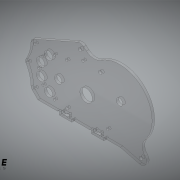
# Autodesk Inventor part: アームフレーム改
Saved by Autodesk Inventor 2020 (Build 240168000, 168)
## iProperties
Created: 2019-12-31
Part Number: アームフレーム改
Material: ポリカーボネート、クリア
Document SubType Name: Modeling
Designer: tanjihayato
Density: 1.2 g/cm^3
Appearance: ポリカーボネート - クリア
Author: tanjihayato
Autodesk Inventor part; units mm, degrees
ref_plane "YZ Plane" through (0, 0, 0) normal (1, 0, 0) x (0, 1, 0)
ref_plane "XZ Plane" through (0, 0, 0) normal (0, 1, 0) x (-1, 0, 0)
ref_plane "XY Plane" through (0, 0, 0) normal (0, 0, 1) x (1, 0, 0)
sketch "スケッチ2" plane through (0, 0, 0) normal (0, 0, 1) x (1, 0, 0)
  circle A0 centre (54.047, 13.5882) radius 4.025
  circle A1 centre (80.4159, -30.3183) radius 2
  circle A2 centre (30.7326, 32.4678) radius 2
  circle A3 centre (3.7003, 45.5208) radius 2
  circle A4 centre (8.8763, 3.8907) radius 7.5
  circle A5 centre (-39.4931, -19.1593) radius 5
  circle A6 centre (-49.0547, -7.5196) radius 5
  circle A7 centre (-49.0547, 7.5438) radius 5
  circle A8 centre (-39.4931, 19.1835) radius 5
  circle A9 centre (-28.0204, 0.0121) radius 4.5
  circle A10 centre (-5.4761, 38.5895) radius 1.5
  circle A11 centre (69.7531, -26.0108) radius 1.5
  circle A12 centre (12.7384, 41.2415) radius 1.5
  circle A13 centre (-56.0504, -23.0135) radius 1.5
  circle A14 centre (-16.1798, -24.0771) radius 1.5
  circle A15 centre (-64.2952, 0.0121) radius 1.5
  circle A16 centre (-56.0504, 23.0377) radius 1.5
  circle A17 centre (-21.4477, 26.0369) radius 1.5
  circle A18 centre (34.0114, -24.0061) radius 1.5
  circle A19 centre (-32.6283, -23.2673) radius 1.3
  circle A20 centre (-46.3578, -15.0513) radius 1.3
  circle A21 centre (-51.7515, 0.0121) radius 1.3
  circle A22 centre (-46.3578, 15.0755) radius 1.3
  circle A23 centre (-32.6283, 23.2915) radius 1.3
  line L0 (-24.5547, -30.1593) -> (-24.5547, -33.1593)
  arc A24 (-26.6547, -33.1593) -> (-24.5547, -33.1593) centre (-25.6047, -33.1593) ccw
  line L1 (-26.6547, -33.1593) -> (-31.4547, -33.1593)
  arc A25 (-33.5547, -33.1593) -> (-31.4547, -33.1593) centre (-32.5047, -33.1593) ccw
  line L2 (-33.5547, -33.1593) -> (-33.5547, -30.1593)
  arc A26 (-31.4547, -30.1593) -> (-33.5547, -30.1593) centre (-32.5047, -30.1593) ccw
  line L3 (-31.4547, -30.1593) -> (-26.6547, -30.1593)
  arc A27 (-24.5547, -30.1593) -> (-26.6547, -30.1593) centre (-25.6047, -30.1593) ccw
  line L4 (13.9305, -30.1593) -> (13.9305, -33.1593)
  arc A28 (11.8305, -33.1593) -> (13.9305, -33.1593) centre (12.8805, -33.1593) ccw
  line L5 (11.8305, -33.1593) -> (7.0305, -33.1593)
  arc A29 (4.9305, -33.1593) -> (7.0305, -33.1593) centre (5.9805, -33.1593) ccw
  line L6 (4.9305, -33.1593) -> (4.9305, -30.1593)
  arc A30 (7.0305, -30.1593) -> (4.9305, -30.1593) centre (5.9805, -30.1593) ccw
  line L7 (7.0305, -30.1593) -> (11.8305, -30.1593)
  arc A31 (13.9305, -30.1593) -> (11.8305, -30.1593) centre (12.8805, -30.1593) ccw
  arc A32 (19.0305, -33.1593) -> (16.9305, -33.1593) centre (17.9805, -33.1593) ccw
  line L8 (19.0305, -33.1593) -> (56.2168, -33.1593)
  line L9 (56.2168, -33.1593) -> (79.2003, -37.212)
  arc A33 (79.2003, -37.212) -> (87.3507, -31.2711) centre (80.4159, -30.3183) ccw
  line L10 (87.3507, -31.2711) -> (92.7831, 8.2659)
  arc A34 (92.7831, 8.2659) -> (29.742, 44.2162) centre (54.047, 13.5882) ccw
  arc A35 (15.9809, 44.3871) -> (29.742, 44.2162) centre (22.9664, 52.7545) ccw
  line L11 (15.9809, 44.3871) -> (8.1864, 50.8943)
  arc A36 (8.1864, 50.8943) -> (0.9804, 51.9708) centre (3.7003, 45.5208) ccw
  line L12 (0.9804, 51.9708) -> (-67.2952, 23.1796)
  line L13 (-67.2952, 23.1796) -> (-67.2952, -18.1327)
  line L14 (-67.2952, -18.1327) -> (-52.2685, -33.1593)
  line L15 (-52.2685, -33.1593) -> (-38.6547, -33.1593)
  arc A37 (-36.5547, -33.1593) -> (-38.6547, -33.1593) centre (-37.6047, -33.1593) ccw
  line L16 (-36.5547, -33.1593) -> (-36.5547, -36.1593)
  line L17 (-36.5547, -36.1593) -> (-21.5547, -36.1593)
  line L18 (-21.5547, -36.1593) -> (-21.5547, -33.1593)
  arc A38 (-19.4547, -33.1593) -> (-21.5547, -33.1593) centre (-20.5047, -33.1593) ccw
  line L19 (-19.4547, -33.1593) -> (-0.1695, -33.1593)
  arc A39 (1.9305, -33.1593) -> (-0.1695, -33.1593) centre (0.8805, -33.1593) ccw
  line L20 (1.9305, -33.1593) -> (1.9305, -36.1593)
  line L21 (1.9305, -36.1593) -> (16.9305, -36.1593)
  line L22 (16.9305, -36.1593) -> (16.9305, -33.1593)
  point P0 (0, 0)
  point P1 (0, 0)
  constraints: 46 end point, 40 centre point, 32 point on circle
sketch "スケッチ1" plane through (0, 0, 0) normal (0, 0, 1) x (1, 0, 0)
  line L0 (-170.6512, -31.4118) -> (202.8656, -31.4118) construction
  circle A0 centre (-14, -17.4118) radius 14 construction
  circle A1 centre (14, -17.4118) radius 14 construction
  circle A2 centre (-28.0204, 0.0121) radius 20.05 construction
  circle A3 centre (-28.0204, 0.0121) radius 5.05 construction
  circle A4 centre (5.5774, 0.3907) radius 28.55 construction
  circle A5 centre (5.5774, 0.3907) radius 10.1 construction
  circle A6 centre (45.6606, 13.5882) radius 32.1 construction
  line L1 (-170.915, -81.4118) -> (490.0044, -81.4118)
  circle A7 centre (-28.0204, 0.0121) radius 22.342 construction
  circle A8 centre (-39.4931, 19.1835) radius 14 construction
  circle A9 centre (-49.0547, 7.5438) radius 14 construction
  circle A10 centre (-49.0547, -7.5196) radius 14 construction
  circle A11 centre (-39.4931, -19.1593) radius 14 construction
  circle A12 centre (5.5774, 0.3907) radius 29.55 construction
  circle A13 centre (45.6606, 13.5882) radius 34.1 construction
  line L2 (-67.2952, 44.8622) -> (-67.2952, -57.3934) construction
  line L3 (-149.4523, -1.6098) -> (-132.6633, -31.6026)
  line L4 (-132.7701, -31.4118) -> (-132.7701, 74.0456)
  circle A14 centre (-11.4931, -19.1593) radius 14 construction
  line L5 (-197.2268, -33.1593) -> (179.6604, -33.1593) construction
  circle A15 centre (45.6606, 13.5882) radius 4.025
  circle A16 centre (45.6606, 13.5882) radius 6
  circle A17 centre (-39.4931, 19.1835) radius 5
  circle A18 centre (-49.0547, 7.5438) radius 5
  circle A19 centre (-49.0547, -7.5196) radius 5
  circle A20 centre (-39.4931, -19.1593) radius 5
  circle A21 centre (-39.4931, 19.1835) radius 8 construction
  circle A22 centre (-49.0547, 7.5438) radius 8 construction
  circle A23 centre (-49.0547, -7.5196) radius 8 construction
  circle A24 centre (-39.4931, -19.1593) radius 8 construction
  circle A25 centre (-28.0204, 0.0121) radius 4.5
  circle A26 centre (5.5774, 0.3907) radius 7.5
  line L6 (-17.5497, 32.3149) -> (-46.3578, 15.0755) construction
  line L7 (-46.3578, 15.0755) -> (-51.7515, 0.0121) construction
  line L8 (-51.7515, 0.0121) -> (-46.3578, -15.0513) construction
  line L9 (-46.3578, -15.0513) -> (-37.9391, -20.0892) construction
  circle A27 centre (-32.6283, 23.2915) radius 1.3
  circle A28 centre (-46.3578, 15.0755) radius 1.3
  circle A29 centre (-51.7515, 0.0121) radius 1.3
  circle A30 centre (-46.3578, -15.0513) radius 1.3
  circle A31 centre (-32.6283, -23.2673) radius 1.3
  line L10 (-67.2952, 23.0074) -> (-67.2952, -18.1327)
  arc A32 (69.4805, -38.9096) -> (76.2418, -27.2762) centre (71.1898, -32.1215) ccw
  arc A33 (2.6419, 49.4236) -> (-4.7411, 50.524) centre (-1.9226, 44.1165) ccw
  line L11 (-52.2685, -33.1593) -> (46.6439, -33.1593)
  line L12 (46.6439, -33.1593) -> (69.4805, -38.9096)
  arc A34 (75.6915, -11.451) -> (23.3358, 45.6882) centre (45.6606, 13.5882) ccw
  line L13 (-4.7411, 50.524) -> (-67.2952, 23.0074)
  circle A35 centre (31.0922, -22.157) radius 4.5 construction
  circle A36 centre (31.0922, -22.157) radius 1.5
  circle A37 centre (-18.0319, 24.9264) radius 4.5 construction
  circle A38 centre (-18.0319, 24.9264) radius 1.5
  circle A39 centre (-56.0504, 23.0377) radius 1.5
  circle A40 centre (-56.0504, 23.0377) radius 3 construction
  circle A41 centre (-56.0504, 23.0377) radius 4.5 construction
  circle A42 centre (-64.2952, 0.0121) radius 1.5
  circle A43 centre (-64.2952, 0.0121) radius 3 construction
  circle A44 centre (-64.2952, 0.0121) radius 4.3311 construction
  line L14 (45.6606, 13.5882) -> (91.8641, 32.6996) construction
  line L15 (91.8641, 32.6996) -> (51.4166, 12.9764) construction
  line L16 (51.4166, 12.9764) -> (22.3463, 32.4678) construction
  line L17 (22.3463, 32.4678) -> (45.6606, 13.5882) construction
  line L18 (91.8641, 32.6996) -> (455.8912, 210.2081)
  line L19 (-183.2789, 162.2213) -> (-183.2789, -125.2315)
  line L20 (516.7211, 155.5913) -> (516.7211, -155.5644)
  circle A45 centre (91.8641, 32.6996) radius 7.25
  line L21 (127.8174, 50.2313) -> (416.2031, 132.8973) construction
  line L22 (224.3644, 77.9066) -> (174.0148, 126.537) construction
  circle A46 centre (-1.9226, 44.1165) radius 4
  circle A47 centre (114.3349, 43.6569) radius 2
  circle A48 centre (127.8174, 50.2313) radius 2
  arc A49 (130.5797, 46.0636) -> (126.2347, 54.9742) centre (127.8174, 50.2313) ccw
  line L23 (130.5797, 46.0636) -> (97.5269, 24.1559)
  line L24 (126.2347, 54.9742) -> (88.6196, 42.4225)
  circle A50 centre (22.3463, 32.4678) radius 2
  circle A51 centre (-17.4731, -24.6708) radius 4.5 construction
  circle A52 centre (-17.4731, -24.6708) radius 1.5
  line L25 (-67.2952, -18.1327) -> (-52.2685, -33.1593)
  circle A53 centre (-56.0504, -23.0135) radius 1.5
  circle A54 centre (-56.0504, -23.0135) radius 3 construction
  circle A55 centre (22.3463, 32.4678) radius 4 construction
  arc A56 (45.9958, 17.0721) -> (45.5027, 10.0918) centre (45.6606, 13.5882) ccw construction
  line L26 (88.9298, 31.4858) -> (92.2801, 35.8476) construction
  line L27 (92.2801, 35.8476) -> (94.3823, 30.7652) construction
  line L28 (94.3823, 30.7652) -> (88.9298, 31.4858) construction
  circle A57 centre (94.3823, 30.7652) radius 1.5
  circle A58 centre (92.2801, 35.8476) radius 1.5
  circle A59 centre (88.9298, 31.4858) radius 1.5
  circle A60 centre (91.8641, 32.6996) radius 6
  arc A61 (96.9465, 25.8864) -> (84.4967, 36.9388) centre (91.8641, 32.6996) ccw
  arc A62 (45.9958, 17.0721) -> (84.4967, 36.9388) centre (49.8265, 56.8883) ccw construction
  arc A63 (45.5027, 10.0918) -> (96.9465, 25.8864) centre (49.1121, 90.0103) ccw construction
  circle A64 centre (45.6606, 13.5882) radius 8.5 construction
  line L29 (88.6151, 40.5541) -> (42.4117, 21.4428) construction
  line L30 (48.9096, 5.7336) -> (95.113, 24.845) construction
  circle A65 centre (71.1898, -32.1215) radius 4
  circle A66 centre (-56.0504, -23.0135) radius 4.5 construction
  line L31 (2.6419, 49.4236) -> (5.9468, 46.5813)
  circle A67 centre (1.6221, 34.2101) radius 1.5
  circle A68 centre (1.6221, 34.2101) radius 4.5 construction
  circle A69 centre (45.6606, 13.5882) radius 50 construction
  circle A70 centre (-1.9226, 44.1165) radius 2
  circle A71 centre (71.1898, -32.1215) radius 2
  circle A72 centre (45.6606, 13.5882) radius 1.5 construction
  circle A73 centre (51.4166, 12.9764) radius 1.5 construction
  circle A74 centre (51.4166, 12.9764) radius 3 construction
  circle A75 centre (51.4166, 12.9764) radius 5 construction
  line L32 (95.251, 23.0253) -> (53.0688, 8.2573) construction
  line L33 (48.7158, 17.1842) -> (86.3274, 41.3256) construction
  arc A76 (88.6196, 42.4225) -> (86.3274, 41.3256) centre (91.8641, 32.6996) ccw
  arc A77 (95.251, 23.0253) -> (97.5269, 24.1559) centre (91.8641, 32.6996) ccw
  circle A78 centre (22.3463, 32.4678) radius 5.025 construction
  circle A79 centre (22.3463, 32.4678) radius 8.025 construction
  circle A80 centre (51.4166, 12.9764) radius 4.025 construction
  circle A81 centre (51.4166, 12.9764) radius 7.025 construction
  line L34 (18.0694, 25.6774) -> (47.6727, 7.0322) construction
  line L35 (46.0495, 17.5091) -> (29.1233, 28.1698) construction
  line L36 (58.3798, 13.9061) -> (60.365, -0.9619) construction
  line L37 (60.365, -0.9619) -> (47.6727, 7.0322) construction
  arc A82 (5.9468, 46.5813) -> (23.3358, 45.6882) centre (15.2178, 57.3607) ccw
  circle A83 centre (5.5774, 0.3907) radius 12.1 construction
  circle A84 centre (-28.0204, 0.0121) radius 20.55 construction
  line L38 (-10.1028, -29.1593) -> (39.2109, -29.1593) construction
  arc A85 (75.6915, -11.451) -> (76.2418, -27.2762) centre (84.8125, -19.056) ccw
  line L39 (-36.5547, -36.1593) -> (-21.5547, -36.1593) projected
  line L40 (1.9305, -36.1593) -> (16.9305, -36.1593) projected
  line L41 (-26.5547, -36.1593) -> (-11.5547, -36.1593)
  line L42 (11.9305, -36.1593) -> (26.9305, -36.1593)
  line L43 (-26.5547, -36.1593) -> (-26.5547, -33.1593)
  line L44 (11.9305, -36.1593) -> (11.9305, -33.1593)
  line L45 (26.9305, -36.1593) -> (26.9305, -33.1593)
  line L46 (-11.5547, -36.1593) -> (-11.5547, -33.1593)
  point P0 (0, 0)
  point P1 (0, 0)
  point P2 (-49.0547, 7.5438)
  point P3 (-49.0547, -7.5196)
  dimension "d0" = 40.1
  dimension "d1" = 10.1
  dimension "d2" = 20.2
  dimension "d3" = 95
  dimension "d4" = 44.684
  dimension "d5" = 28
  dimension "d6" = 28
  dimension "d7" = 28
  dimension "d8" = 28
  dimension "d9" = 1
  dimension "d10" = 2
  dimension "d11" = 8.05
  dimension "d12" = 12
  dimension "d13" = 10
  dimension "d14" = 10
  dimension "d15" = 10
  dimension "d16" = 10
  dimension "d17" = 3
  dimension "d18" = 3
  dimension "d19" = 3
  dimension "d20" = 3
  dimension "d21" = 9
  dimension "d22" = 15
  dimension "d23" = 2.6
  dimension "d24" = 2.6
  dimension "d25" = 2.6
  dimension "d26" = 2.6
  dimension "d27" = 2.6
  dimension "d28" = 5
  dimension "d29" = 9
  dimension "d30" = 3
  dimension "d31" = 9
  dimension "d32" = 3
  dimension "d33" = 3
  dimension "d34" = 6
  dimension "d35" = 9
  dimension "d36" = 3
  dimension "d37" = 6
  dimension "d38" = 50
  dimension "d39" = 45
  dimension "d40" = 35
  dimension "d41" = 30
  dimension "d42" = 39
  dimension "d43" = 700
  dimension "d44" = 14.5
  dimension "d45" = 300
  dimension "d46" = 10
  dimension "d47" = 70
  dimension "d48" = 120
  dimension "d49" = 140
  dimension "d50" = 8
  dimension "d51" = 4
  dimension "d52" = 4
  dimension "d53" = 15
  dimension "d54" = 25
  dimension "d55" = 10
  dimension "d56" = 4
  dimension "d57" = 9
  dimension "d58" = 3
  dimension "d59" = 3
  dimension "d60" = 6
  dimension "d61" = 45
  dimension "d62" = 8
  dimension "d63" = 7
  constraints: 90 end point, 83 centre point, 53 tangent, 44 coincident, 41 point on circle, 17 point on line, 7 vertical, 4 horizontal, 4 midpoint, 2 collinear, 1 parallel, 1 perpendicular, 1 vertical alignment, 18 other
  measures "d0" diameter of A2
  measures "d1" diameter of A3
  measures "d2" diameter of A5
  measures "d3" distance from line of L1 A6.centre
  measures "d4" diameter of A7
  measures "d5" diameter of A8
  measures "d6" diameter of A9
  measures "d7" diameter of A10
  measures "d8" diameter of A11
  measures "d9" radial gap between concentric circles of A4 A12
  measures "d10" radial gap between concentric circles of A6 A13
  measures "d11" diameter of A15
  measures "d12" diameter of A16
  measures "d13" diameter of A17
  measures "d14" diameter of A18
  measures "d15" diameter of A19
  measures "d16" diameter of A20
  measures "d17" radial gap between concentric circles of A17 A21
  measures "d21" diameter of A25
  measures "d22" diameter of A26
  measures "d23" diameter of A27
  measures "d24" diameter of A28
  measures "d25" diameter of A29
  measures "d26" diameter of A30
  measures "d27" diameter of A31
  measures "d28" radial gap between concentric circles of A13 A34
  measures "d29" diameter of A35
  measures "d30" diameter of A36
  measures "d31" diameter of A37
  measures "d32" diameter of A38
  measures "d33" diameter of A39
  measures "d34" diameter of A40
  measures "d35" diameter of A41
  measures "d36" diameter of A42
  measures "d37" diameter of A43
  measures "d38" distance of L14.start L14.end
  measures "d39" distance of L14.end L15.end
  measures "d40" distance of L15.end L16.end
  measures "d41" distance of L16.end L14.start
  measures "d42" angle of L0 L17
  measures "d43" distance between parallel lines of L20 L19
  measures "d44" diameter of A45
  measures "d45" distance of L21.start L21.end
  measures "d46" angle of L18 L21
  measures "d47" distance of L22.start L22.end
  measures "d48" angle of L21 L22
  measures "d49" distance of L14.end L22.start
  measures "d50" diameter of A46
  measures "d51" diameter of A47
  measures "d52" diameter of A48
  measures "d53" distance of L21.start A47.centre
  measures "d54" distance of A47.centre A45.centre
  measures "d55" diameter of A49
  measures "d56" diameter of A50
  measures "d57" diameter of A51
  measures "d58" diameter of A52
  measures "d59" diameter of A53
  measures "d60" diameter of A54
  measures "d61" angle of L5 L25
  measures "d62" diameter of A55
  measures "d63" diameter of A56
extrude "押し出し1" add sketch "スケッチ1" along normal blind 3 contours A16 | L13 A33 L31 A82 A34 A85 A32 L12 L11 L25 L10 | L11 L46 L41 L39 L43 | L11 L45 L42 L40 L44 | A46 | A65
sketch "スケッチ3" plane through (0, 0, 3) normal (0, 0, 1) x (1, 0, 0)
  line L0 (-52.2685, -33.1593) -> (-26.5547, -33.1593) projected
  line L1 (-26.5547, -33.1593) -> (-26.5547, -36.1593) projected
  line L2 (-26.5547, -36.1593) -> (-11.5547, -36.1593) projected
  line L3 (-11.5547, -36.1593) -> (-11.5547, -33.1593) projected
  line L4 (-11.5547, -33.1593) -> (11.9305, -33.1593) projected
  line L5 (11.9305, -33.1593) -> (11.9305, -36.1593) projected
  line L6 (11.9305, -36.1593) -> (26.9305, -36.1593) projected
  line L7 (26.9305, -36.1593) -> (26.9305, -33.1593) projected
  line L8 (26.9305, -33.1593) -> (46.6439, -33.1593) projected
  line L9 (46.6439, -33.1593) -> (69.4805, -38.9096) projected
  arc A0 (69.4805, -38.9096) -> (76.2418, -27.2762) centre (71.1898, -32.1215) ccw projected
  arc A1 (75.6915, -11.451) -> (76.2418, -27.2762) centre (84.8125, -19.056) ccw projected
  arc A2 (75.6915, -11.451) -> (23.3358, 45.6882) centre (45.6606, 13.5882) ccw projected
  arc A3 (5.9468, 46.5813) -> (23.3358, 45.6882) centre (15.2178, 57.3607) ccw projected
  line L10 (5.9468, 46.5813) -> (2.6419, 49.4236) projected
  arc A4 (2.6419, 49.4236) -> (-4.7411, 50.524) centre (-1.9226, 44.1165) ccw projected
  line L11 (-4.7411, 50.524) -> (-67.2952, 23.0074) projected
  line L12 (-67.2952, 23.0074) -> (-67.2952, -18.1327) projected
  line L13 (-67.2952, -18.1327) -> (-52.2685, -33.1593) projected
  circle A5 centre (-1.9226, 44.1165) radius 2 projected
  circle A6 centre (45.6606, 13.5882) radius 4.025 projected
  circle A7 centre (1.6221, 34.2101) radius 1.5 projected
  circle A8 centre (31.0922, -22.157) radius 1.5 projected
  circle A9 centre (-46.3578, -15.0513) radius 1.3 projected
  circle A10 centre (-46.3578, 15.0755) radius 1.3 projected
  circle A11 centre (5.5774, 0.3907) radius 7.5 projected
  circle A12 centre (-28.0204, 0.0121) radius 4.5 projected
  circle A13 centre (-39.4931, -19.1593) radius 5 projected
  circle A14 centre (-49.0547, -7.5196) radius 5 projected
  circle A15 centre (-49.0547, 7.5438) radius 5 projected
  circle A16 centre (-51.7515, 0.0121) radius 1.3 projected
  circle A17 centre (-32.6283, -23.2673) radius 1.3 projected
  circle A18 centre (-64.2952, 0.0121) radius 1.5 projected
  circle A19 centre (-17.4731, -24.6708) radius 1.5 projected
  circle A20 centre (22.3463, 32.4678) radius 2 projected
  circle A21 centre (-18.0319, 24.9264) radius 1.5 projected
  circle A22 centre (-56.0504, 23.0377) radius 1.5 projected
  circle A23 centre (-32.6283, 23.2915) radius 1.3 projected
  circle A24 centre (-56.0504, -23.0135) radius 1.5 projected
  circle A25 centre (-39.4931, 19.1835) radius 5 projected
  circle A26 centre (71.1898, -32.1215) radius 2 projected
  circle A27 centre (-56.0504, 23.0377) radius 4.5
  circle A28 centre (-64.2952, 0.0121) radius 3
  circle A29 centre (-56.0504, -23.0135) radius 4.5
  arc A30 (-66.8752, 1.5429) -> (-60.5479, 23.1875) centre (-105.8992, 24.6978) ccw
  arc A31 (-60.5479, -23.1633) -> (-66.8752, -1.5188) centre (-105.8992, -24.6736) ccw
  circle A32 centre (-49.0547, -7.5196) radius 14 construction
  circle A33 centre (-49.0547, 7.5438) radius 14 construction
  line L14 (-23.5547, -30.1593) -> (-14.5547, -30.1593)
  line L15 (-14.5547, -30.1593) -> (-14.5547, -33.1593)
  line L16 (-14.5547, -33.1593) -> (-23.5547, -33.1593)
  line L17 (-23.5547, -33.1593) -> (-23.5547, -30.1593)
  line L18 (14.9305, -30.1593) -> (23.9305, -30.1593)
  line L19 (23.9305, -30.1593) -> (23.9305, -33.1593)
  line L20 (23.9305, -33.1593) -> (14.9305, -33.1593)
  line L21 (14.9305, -33.1593) -> (14.9305, -30.1593)
  line L22 (-11.5547, -33.1593) -> (11.9305, -33.1593) projected
  circle A34 centre (-22.5047, -30.1593) radius 1.05
  circle A35 centre (-15.6047, -30.1593) radius 1.05
  circle A36 centre (-15.6047, -33.1593) radius 1.05
  circle A37 centre (-22.5047, -33.1593) radius 1.05
  circle A38 centre (15.9805, -30.1593) radius 1.05
  circle A39 centre (22.8805, -30.1593) radius 1.05
  circle A40 centre (15.9805, -33.1593) radius 1.05
  circle A41 centre (22.8805, -33.1593) radius 1.05
  circle A42 centre (10.8805, -33.1593) radius 1.05
  circle A43 centre (27.9805, -33.1593) radius 1.05
  circle A44 centre (-10.5047, -33.1593) radius 1.05
  line L23 (-52.2685, -33.1593) -> (-26.5547, -33.1593) projected
  circle A45 centre (-27.6047, -33.1593) radius 1.05
  line L24 (-26.5547, -33.1593) -> (-26.5547, -36.1593) projected
  line L25 (-11.5547, -36.1593) -> (-11.5547, -33.1593) projected
  line L26 (11.9305, -33.1593) -> (11.9305, -36.1593) projected
  line L27 (26.9305, -36.1593) -> (26.9305, -33.1593) projected
  circle A46 centre (45.6606, 13.5882) radius 6
  point P0 (0, 0)
  point P1 (17.0305, -33.1593)
  point P2 (21.8305, -33.1593)
  point P3 (21.8305, -30.1593)
  point P4 (17.0305, -30.1593)
  point P5 (-16.6547, -30.1593)
  point P6 (-21.4547, -30.1593)
  point P7 (-21.4547, -33.1593)
  point P8 (-16.6547, -33.1593)
  point P9 (-67.2952, 0.0121)
  point P10 (-59.2324, -26.1955)
  point P11 (-57.8623, 27.1568)
  dimension "d108" = 9
  dimension "d109" = 3
  dimension "d110" = 9
  dimension "d111" = 3
  dimension "d112" = 3
  dimension "d113" = 3
  dimension "d114" = 2.1
  dimension "d115" = 2.1
  dimension "d116" = 2.1
  dimension "d117" = 2.1
  dimension "d118" = 2.1
  dimension "d119" = 2.1
  dimension "d120" = 2.1
  dimension "d121" = 2.1
  dimension "d122" = 2.1
  dimension "d123" = 2.1
  dimension "d124" = 2.1
  dimension "d125" = 2.1
  dimension "d126" = 12
  constraints: 17 tangent, 16 centre point, 16 end point, 13 point on line, 6 point on circle, 4 coincident, 4 parallel, 2 horizontal, 2 perpendicular, 1 collinear, 10 other
  measures "d108" distance of L15.end L16.end
  measures "d109" distance of L14.end L15.end
  measures "d110" distance of L19.end L20.end
  measures "d111" distance of L18.end L19.end
  measures "d112" distance between parallel lines of L1 L17
  measures "d113" distance between parallel lines of L5 L21
  measures "d114" diameter of A34
  measures "d115" diameter of A35
  measures "d116" diameter of A36
  measures "d117" diameter of A37
  measures "d118" diameter of A38
  measures "d119" diameter of A39
  measures "d120" diameter of A40
  measures "d121" diameter of A41
  measures "d122" diameter of A42
  measures "d123" diameter of A43
  measures "d124" diameter of A44
  measures "d125" diameter of A45
  measures "d126" diameter of A46
extrude "押し出し2" cut sketch "スケッチ3" against normal blind 3 contours A45 L0 | L0 A45 | L13 L12 A28 A31 A29 | L12 L11 A27 A30 A28 | A44 L4 | L4 A44 | A42 L4 | L4 A42 | A43 L8 | L8 A43 | A34 L14 | A34 L14 A35 L15 A36 L16 A37 L17 | L14 A34 | A37 L16 | L16 A37 | A35 L14 | L14 A35 | A36 L16 | L16 A36 | A38 L18 | A38 L18 A39 L19 A41 L20 A40 L21 | L18 A38 | A40 L20 | L20 A40 | A39 L18 | L18 A39 | A41 L20 | L20 A41
